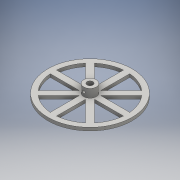
# Autodesk Inventor part: Part3
Saved by Autodesk Inventor 2016 SP1 (Build 200210100, 210)
## iProperties
Created: 2018-04-30
Part Number: Part3
Material: 一般
Document SubType Name: Modeling
Designer: kobay
Density: 1 g/cm^3
Appearance: 既定
Author: kobay
Autodesk Inventor part; units mm, degrees
ref_plane "YZ Plane" through (0, 0, 0) normal (1, 0, 0) x (0, 1, 0)
ref_plane "XY Plane" through (0, 0, 0) normal (0, 0, 1) x (1, 0, 0)
sketch "スケッチ1" plane through (0, 0, 0) normal (0, 0, 1) x (1, 0, 0)
  circle A0 centre (0, 0) radius 40
  circle A1 centre (0, 0) radius 2.5
  dimension "d0" = 80
  dimension "d1" = 5
  constraints: 2 centre point, 2 coincident
  measures "d0" diameter of A0
  measures "d1" diameter of A1
extrude "押し出し1" add sketch "スケッチ1" along normal blind 3
sketch "スケッチ2" plane through (0, 0, 3) normal (0, 0, 1) x (1, 0, 0)
  circle A0 centre (0, 0) radius 8
  circle A1 centre (0, 0) radius 2.5 projected
  circle A2 centre (0, 0) radius 35
  line L0 (3, 34.8712) -> (3, 7.4162)
  line L1 (-3, 7.4162) -> (-3, 34.8712)
  line L2 (-7.3654, 3.1227) -> (-26.779, 22.5363)
  line L3 (-22.5363, 26.779) -> (-3.1227, 7.3654)
  circle A3 centre (0, 0) radius 35
  circle A4 centre (0, 0) radius 8
  line L4 (-7.4162, -3) -> (-34.8712, -3)
  line L5 (-34.8712, 3) -> (-7.4162, 3)
  circle A5 centre (0, 0) radius 35
  circle A6 centre (0, 0) radius 8
  line L6 (-3.1227, -7.3654) -> (-22.5363, -26.779)
  line L7 (-26.779, -22.5363) -> (-7.3654, -3.1227)
  circle A7 centre (0, 0) radius 35
  circle A8 centre (0, 0) radius 8
  line L8 (3, -7.4162) -> (3, -34.8712)
  line L9 (-3, -34.8712) -> (-3, -7.4162)
  circle A9 centre (0, 0) radius 35
  circle A10 centre (0, 0) radius 8
  line L10 (7.3654, -3.1227) -> (26.779, -22.5363)
  line L11 (22.5363, -26.779) -> (3.1227, -7.3654)
  circle A11 centre (0, 0) radius 35
  circle A12 centre (0, 0) radius 8
  line L12 (7.4162, 3) -> (34.8712, 3)
  line L13 (34.8712, -3) -> (7.4162, -3)
  circle A13 centre (0, 0) radius 35
  circle A14 centre (0, 0) radius 8
  line L14 (3.1227, 7.3654) -> (22.5363, 26.779)
  line L15 (26.779, 22.5363) -> (7.3654, 3.1227)
  circle A15 centre (0, 0) radius 35
  circle A16 centre (0, 0) radius 8
  dimension "d4" = 16
  dimension "d5" = 70
  dimension "d6" = 3
  dimension "d7" = 6
  dimension "d10" = 360
  constraints: 32 end point, 32 point on circle, 16 centre point, 4 coincident, 1 parallel, 79 other
  measures "d4" diameter of A0
  measures "d5" diameter of A2
  measures "d6" distance from line of point (0, 0) L1
  measures "d7" distance between parallel lines of L0 L1
extrude "押し出し2" cut sketch "スケッチ2" against normal blind 5 contours A0 L15 A2 L12 | L13 A2 L10 A0 | A0 L0 A2 L14 | L11 A2 L8 A0 | A0 L3 A2 L1 | L9 A2 L6 A0 | A0 L5 A2 L2 | L7 A2 L4 A0
sketch "スケッチ3" plane through (0, 0, 3) normal (0, 0, 1) x (1, 0, 0)
  circle A0 centre (0, 0) radius 2.5 projected
  circle A1 centre (0, 0) radius 2.5
  circle A2 centre (0, 0) radius 6
  dimension "d14" = 12
  constraints: 2 centre point, 2 coincident
  measures "d14" diameter of A2
extrude "押し出し3" add sketch "スケッチ3" along normal blind 8
ref_plane "作業平面1" through (0, 0, 0) normal (0, 1, 0) x (-1, 0, 0)
sketch "スケッチ4" plane through (0, 0, 0) normal (0, 1, 0) x (-1, 0, 0)
  circle A0 centre (0, 7) radius 1.25
  line L0 (40, 3) -> (-40, 3) projected
  point P0 (0, 0)
  dimension "d18" = 2.5
  dimension "d19" = 4
  constraints: 1 centre point
  measures "d18" diameter of A0
  measures "d19" distance from line of L0 A0.centre
extrude "押し出し4" cut sketch "スケッチ4" along normal mid plane 15
sketch "スケッチ5" plane through (0, 0, 11) normal (0, 0, 1) x (1, 0, 0)
  circle A0 centre (0, 0) radius 2.8
  dimension "d22" = 5.6
  constraints: 1 centre point, 1 coincident
  measures "d22" diameter of A0
extrude "押し出し5" cut sketch "スケッチ5" against normal blind 20
